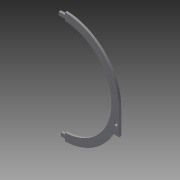
# Autodesk Inventor part: TopmaleHoopSection_v2
Saved by Autodesk Inventor 2013 (Build 170138000, 138)
## iProperties
Created: 2013-01-17
Part Number: TopmaleHoopSection_v2
Material: Generic
Document SubType Name: Modeling
Designer: twsass
Density: 1 g/cm^3
Author: twsass
Autodesk Inventor part; units mm, degrees
ref_plane "YZ Plane" through (0, 0, 0) normal (1, 0, 0) x (0, 1, 0)
ref_plane "XZ Plane" through (0, 0, 0) normal (0, 1, 0) x (-1, 0, 0)
ref_plane "XY Plane" through (0, 0, 0) normal (0, 0, 1) x (1, 0, 0)
sketch "Sketch1" plane through (0, 0, 0) normal (0, 0, 1) x (1, 0, 0)
  circle A0 centre (0, 0) radius 146.05
  arc A1 (168.91, 0) -> (150.7453, -76.2) centre (0, 0) ccw
  line L0 (6.35, -145.9119) -> (6.35, -168.7906)
  circle A2 centre (-157.48, 0) radius 3.175
  line L1 (6.35, -145.9119) -> (6.35, -150.9919)
  line L2 (6.35, -150.9919) -> (-6.35, -150.9919)
  line L3 (-6.35, -150.9919) -> (-6.35, -161.1519)
  line L4 (-6.35, -161.1519) -> (6.35, -161.1519)
  line L5 (6.35, -150.9919) -> (6.35, -161.1519)
  line L6 (6.35, 145.9119) -> (6.35, 168.7906)
  line L7 (0, 0) -> (0, 200.5264) construction
  line L8 (6.35, 145.9119) -> (6.35, 150.9919) construction
  line L9 (6.35, 150.9919) -> (-12.7, 150.9919)
  line L10 (-12.7, 150.9919) -> (-12.7, 161.1519)
  line L11 (-12.7, 161.1519) -> (6.35, 161.1519)
  line L12 (0, -146.05) -> (0, 0) construction
  line L13 (168.91, 0) -> (168.91, -76.2)
  line L14 (168.91, -76.2) -> (150.7453, -76.2)
  line L15 (0, 0) -> (0, -47.2694) construction
  line L16 (0, -47.2694) -> (158.75, -47.2694) construction
  line L17 (158.75, -42.5069) -> (163.83, -42.5069)
  line L18 (163.83, -42.5069) -> (163.83, -52.0319)
  line L19 (163.83, -52.0319) -> (153.67, -52.0319)
  line L20 (153.67, -52.0319) -> (153.67, -42.5069)
  line L21 (153.67, -42.5069) -> (158.75, -42.5069)
  point P0 (0.0447, 168.91)
  point P1 (6.3947, 145.9099)
  dimension "d51" = 292.1
  dimension "d52" = 337.82
  dimension "d58" = 5.08
  dimension "d59" = 12.7
  dimension "d60" = 10.16
  dimension "d72" = 6.35
  dimension "d73" = 5.08
  dimension "d75" = 19.05
  dimension "d76" = 10.16
  dimension "d77" = 6.35
  dimension "d82" = 76.2
  dimension "d86" = 47.2694
  dimension "d87" = 158.75
  dimension "d89" = 4.7625
  dimension "d90" = 5.08
  dimension "d91" = 9.525
  dimension "d92" = 10.16
  dimension "d93" = 4.7625
  constraints: 44 end point, 9 point on circle, 8 perpendicular, 4 parallel, 3 centre point, 3 point on line, 1 coincident, 1 collinear, 1 tangent, 1 vertical
  measures "d51" diameter of A0
  measures "d52" diameter of A1
  measures "d58" distance of L0.start L1.end
  measures "d59" distance of L1.end L2.end
  measures "d60" distance of L2.end L3.end
  measures "d72" distance between parallel lines of L6 L7
  measures "d73" distance of L6.start L8.end
  measures "d75" distance of L8.end L9.end
  measures "d76" distance of L9.end L10.end
  measures "d77" distance between parallel lines of L12 L1
  measures "d82" distance of L13.start L13.end
  measures "d86" distance of L7.start L15.end
  measures "d87" distance of L15.end L16.end
  measures "d89" distance of L16.end L17.start
  measures "d90" distance of L17.start L17.end
  measures "d91" distance of L17.end L18.end
  measures "d92" distance of L18.end L19.end
  measures "d93" distance between parallel lines of L16 L21
extrude "Extrusion16" add sketch "Sketch1" along normal blind 6.35 contours A0 L6 A1 L13 L14 L0 | L9 L10 L11 L6 | L0 L4 L3 L2
body "Solid9"
